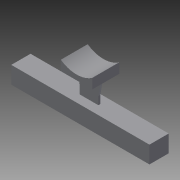
# Autodesk Inventor part: SLIDE_POTENTIOMETER
Saved by Autodesk Inventor 2015 (Build 190159000, 159)
## iProperties
Created: 2015-02-07
Part Number: SLIDE_POTENTIOMETER
Material: Generic
Document SubType Name: Modeling
Designer: lucanao16
Density: 1 g/cm^3
Appearance: Default
Author: lucanao16
Autodesk Inventor part; units mm, degrees
ref_plane "YZ Plane" through (0, 0, 0) normal (1, 0, 0) x (0, 1, 0)
ref_plane "XZ Plane" through (0, 0, 0) normal (0, 1, 0) x (-1, 0, 0)
ref_plane "XY Plane" through (0, 0, 0) normal (0, 0, 1) x (1, 0, 0)
sketch "Sketch1" plane through (0, 0, 0) normal (0, 1, 0) x (-1, 0, 0)
  line L0 (0, 0) -> (88.138, 0)
  line L1 (88.138, 0) -> (88.138, -12.2936)
  line L2 (88.138, -12.2936) -> (0, -12.2936)
  line L3 (0, -12.2936) -> (0, 0)
  dimension "d0" = 88.138
  dimension "d1" = 12.2936
  constraints: 8 end point, 2 parallel, 1 horizontal, 1 perpendicular
  measures "d0" distance of L1.end L2.end
  measures "d1" distance of L0.end L1.end
extrude "Extrusion1" add sketch "Sketch1" along normal blind 10.922
sketch "Sketch2" plane through (0, 10.922, 0) normal (0, 1, 0) x (1, 0, 0)
  line L0 (-88.138, 12.2936) -> (-88.138, 0) projected
  line L1 (0, 0) -> (0, 12.2936) projected
  line L2 (-50.038, 6.7818) -> (-38.1, 6.7818)
  line L3 (-38.1, 6.7818) -> (-38.1, 5.5118)
  line L4 (-38.1, 5.5118) -> (-50.038, 5.5118)
  line L5 (-50.038, 5.5118) -> (-50.038, 6.7818)
  dimension "d7" = 11.938
  dimension "d8" = 1.27
  constraints: 8 end point, 2 parallel, 1 horizontal, 1 perpendicular
  measures "d7" distance of L3.end L4.end
  measures "d8" distance of L2.end L3.end
extrude "Extrusion2" add sketch "Sketch2" along normal blind 5.08
sketch "Sketch4" plane through (-50.038, 10.922, -5.5118) normal (0, 0, 1) x (1, 0, 0)
  line L0 (0, 5.08) -> (11.938, 5.08)
  line L1 (11.938, 5.08) -> (0, 5.08) projected
  line L2 (11.938, 5.08) -> (13.6399, 14.732)
  line L3 (11.938, 5.08) -> (21.7389, 5.08) construction
  line L4 (0, 5.08) -> (-1.7019, 14.732)
  line L5 (0, 5.08) -> (9.8009, 5.08) construction
  line L6 (-1.7019, 14.732) -> (13.6399, 14.732)
  point P0 (50.038, -10.922)
  dimension "d12" = 80
  dimension "d13" = 100
  constraints: 12 end point, 3 horizontal, 2 equal length, 1 collinear
  measures "d12" angle of L3 L2
  measures "d13" angle of L5 L4
extrude "Extrusion3" add sketch "Sketch4" against normal blind 1.27
sketch "Sketch5" plane through (-51.7399, 25.654, -5.5118) normal (0, 1, 0) x (1, 0, 0)
  line L0 (15.3418, 0) -> (0, 0) projected
  line L1 (15.3418, 0) -> (15.3418, 1.27) projected
  line L2 (0, 1.27) -> (15.3418, 1.27) projected
  line L3 (0, 0) -> (0, 1.27) projected
  line L4 (-2.3621, 0.635) -> (17.7039, 0.635)
  line L5 (-2.3621, 9.2075) -> (17.7039, 9.2075)
  line L6 (17.7039, 9.2075) -> (17.7039, -7.9375)
  line L7 (17.7039, -7.9375) -> (-2.3621, -7.9375)
  line L8 (-2.3621, -7.9375) -> (-2.3621, 9.2075)
  point P0 (51.7399, -5.5118)
  dimension "d19" = 20.066
  dimension "d21" = 17.145
  dimension "d22" = 8.5725
  dimension "d23" = 0.635
  constraints: 10 end point, 2 parallel, 1 horizontal, 1 perpendicular
  measures "d19" distance of L4.start L4.end
  measures "d21" distance between parallel lines of L7 L5
  measures "d22" distance between parallel lines of L7 L4
  measures "d23" distance between parallel lines of L4 L2
extrude "Extrusion4" add sketch "Sketch5" along normal blind 6.35
sketch "Sketch6" plane through (-54.102, 25.654, 2.4257) normal (0, 0, 1) x (1, 0, 0)
  arc A0 (0, 6.35) -> (20.066, 6.35) centre (10.033, 20.6146) ccw
  line L0 (0, 6.35) -> (20.066, 6.35)
  point P0 (54.102, -25.654)
  constraints: 2 end point, 2 point on circle, 1 centre point, 1 horizontal
extrude "Extrusion5" cut sketch "Sketch6" against normal blind 20.32
body "Solid1"
